Autodesk Fusion 360 part; units mm, degrees
note: some values were not read from the file. Chosen so that the rebuilt part matches the saved one: which face or edge a step refers to. Set by a fixed rule: which sketch regions a step uses; the direction of a hole.
(part 4 of 4)
sketch "Sketch157" plane through (150, 0, 0) normal (-1, 0, 0) x (0, -1, 0)
  line L0 (0, 69) -> (10, 69)
  line L1 (10, 69) -> (10, 66)
  line L2 (10, 66) -> (0, 66)
  line L3 (0, 66) -> (0, 0)
  line L4 (0, 0) -> (45, 0)
  line L5 (45, 0) -> (45, 66)
  line L6 (45, 66) -> (35, 66)
  line L7 (35, 66) -> (35, 69)
  line L8 (35, 69) -> (45, 69)
  line L9 (45, 69) -> (45, 75)
  line L10 (45, 75) -> (34, 75)
  line L11 (34, 75) -> (34, 80)
  line L12 (34, 80) -> (11, 80)
  line L13 (11, 80) -> (11, 75)
  line L14 (11, 75) -> (0, 75)
  line L15 (0, 75) -> (0, 69)
  line L16 (15, 33) -> (30, 33)
  line L17 (30, 33) -> (30, 27)
  line L18 (30, 27) -> (15, 27)
  line L19 (15, 27) -> (15, 33)
  circle A0 centre (17.9, 30) radius 1.5
  circle A1 centre (27.1, 30) radius 1.5
  dimension "d1193" = 27
  dimension "d1194" = 3
  dimension "d1195" = 3
  dimension "d1196" = 9.2
  dimension "d1197" = 3
  dimension "d1198" = 15
  dimension "d1199" = 2.9
  dimension "d1200" = 6
  constraint horizontal L16
  constraint vertical L17
  constraint horizontal L18
  constraint vertical L19
  measures "d1193" distance of L4 L18
  measures "d1194" diameter of A0
  measures "d1195" diameter of A1
  measures "d1196" distance of A0.centre A1.centre
  measures "d1197" distance of L18 A0.centre
  measures "d1198" distance of L16.start L16.end
  measures "d1199" distance of L19 A0.centre
  measures "d1200" distance of L16.start L18.end
extrude "Extrude200" add sketch "Sketch157" along normal blind 10 contours L16 L17 L18 L19 bodies 6
extrude "Extrude201" cut sketch "Sketch157" against normal blind 78.085 contours A0 | A1 bodies 6
sketch "Sketch158" plane through (170, 0, 0) normal (1, 0, 0) x (0, 1, 0)
  circle A0 centre (-17.9, 30) radius 1.5
  circle A1 centre (-27.1, 30) radius 1.5
  line L0 (0, 47) -> (-45, 47)
  line L1 (-45, 47) -> (-45, 10)
  line L2 (-45, 10) -> (0, 10)
  line L3 (0, 10) -> (0, 47)
  circle A2 centre (-27.1, 30) radius 3.5
  circle A3 centre (-17.9, 30) radius 3.5
  dimension "d1205" = 7
  dimension "d1206" = 7
  constraint concentric A1 A2
  constraint concentric A0 A3
  measures "d1205" diameter of A2
  measures "d1206" diameter of A3
extrude "Extrude202" cut sketch "Sketch158" against normal blind 3 contours A2 | A3 bodies 6
extrude "Extrude203" add 1 faces at (-154.4778, 172, 27.586) along direction (0, -1, 0) blind 2.2 on bodies 1 bodies 1
sketch "Sketch159" plane through (0, 0, 120) normal (0, 0, 1) x (-1, 0, 0)
  line L0 (175, -164.8202) -> (171.994, -164.8202)
  line L1 (171.994, -164.8202) -> (171.994, -165.8202)
  line L2 (171.994, -165.8202) -> (169.294, -165.8202)
  line L3 (169.294, -165.8202) -> (169.294, -164.8202)
  line L4 (169.294, -164.8202) -> (160, -164.8202)
  line L5 (160, -164.8202) -> (160, -174.8202)
  line L6 (160, -174.8202) -> (175, -174.8202)
  line L7 (175, -174.8202) -> (175, -164.8202)
  circle A0 centre (163.5, -171.3202) radius 1.5
  circle A1 centre (163.5, -108.3202) radius 1.5
  line L8 (175, -104.8202) -> (160, -104.8202)
  line L9 (160, -104.8202) -> (160, -114.8202)
  dimension "d1211" = 3
  dimension "d1212" = 3.5
  dimension "d1213" = 3.5
  dimension "d1214" = 3
  dimension "d1215" = 3.5
  dimension "d1216" = 3.5
  measures "d1211" diameter of A0
  measures "d1212" distance of L5 A0.centre
  measures "d1213" distance of L6 A0.centre
  measures "d1214" diameter of A1
  measures "d1215" distance of A1.centre L8
  measures "d1216" distance of A1.centre L9
extrude "Extrude204" cut sketch "Sketch159" against normal blind 35 contours A0 | A1 bodies 1
extrude "Extrude205" cut sketch "Sketch155" against normal blind 7 contours L10 L21 L22 L23 L24 | L7 L17 L18 L19 L20 bodies 1
sketch "Sketch160" plane through (0, 0, 15) normal (0, 0, 1) x (-1, 0, 0)
  line L0 (175, 4.7712) -> (25, 4.7712)
  line L1 (25, 4.7712) -> (25, 0)
  line L2 (25, 0) -> (-15, 0)
  line L3 (-15, 0) -> (-15, -30)
  line L4 (-15, -30) -> (190, -30)
  line L5 (190, -30) -> (190, -5)
  line L6 (190, -5) -> (176, -5)
  arc A0 (175, -4) -> (176, -5) centre (175, -5) ccw
  line L7 (175, -4) -> (175, 4.7712)
  circle A1 centre (120, -15) radius 2.5
  circle A2 centre (120, 75) radius 2.5
  circle A3 centre (55, 75) radius 2.5
  circle A4 centre (55, -15) radius 2.5
  circle A5 centre (120, 75) radius 5
  circle A6 centre (120, -15) radius 5
  circle A7 centre (55, -15) radius 5
  circle A8 centre (55, 75) radius 5
  line L8 (190, -30) -> (190, -10)
  line L9 (190, 65) -> (190, 90)
  line L10 (-15, 90) -> (-15, 60)
  line L11 (190, 90) -> (-15, 90)
  line L12 (-15, -30) -> (190, -30)
  dimension "d1227" = 5
  dimension "d1228" = 5
  dimension "d1229" = 5
  dimension "d1230" = 5
  dimension "d1235" = 70
  dimension "d1236" = 70
  dimension "d1237" = 70
  dimension "d1238" = 70
  dimension "d1239" = 15
  dimension "d1240" = 15
  dimension "d1241" = 15
  dimension "d1242" = 15
  constraint concentric A2 A5
  constraint concentric A1 A6
  constraint concentric A4 A7
  constraint concentric A3 A8
  measures "d1227" diameter of A1
  measures "d1228" diameter of A2
  measures "d1229" diameter of A3
  measures "d1230" diameter of A4
  measures "d1235" distance of A1.centre L8
  measures "d1236" distance of L3 A4.centre
  measures "d1237" distance of A2.centre L9
  measures "d1238" distance of A3.centre L10
  measures "d1239" distance of A3.centre L11
  measures "d1240" distance of A2.centre L11
  measures "d1241" distance of A1.centre L12
  measures "d1242" distance of A4.centre L12
extrude "Extrude206" cut sketch "Sketch160" against normal blind 22.636 contours A1 | A2 | A3 | A4 bodies 2
extrude "Extrude207" cut sketch "Sketch160" against normal blind 10 contours A5 | A6 | A7 | A8 bodies 2
sketch "Sketch161" plane through (0, 0, 0) normal (0, 0, 1) x (1, 0, 0)
  line L0 (-75, -100) -> (-160, -100)
  line L1 (-160, -100) -> (-160, -220)
  line L2 (-160, -220) -> (-75, -220)
  line L3 (-75, -220) -> (-75, -100)
  circle A0 centre (-150, -115) radius 2.5
  circle A1 centre (-85, -115) radius 2.5
  circle A2 centre (-150, -205) radius 2.5
  circle A3 centre (-85, -205) radius 2.5
  dimension "d1243" = 85
  dimension "d1244" = 120
  dimension "d1245" = 5
  dimension "d1246" = 5
  dimension "d1247" = 65
  dimension "d1248" = 5
  dimension "d1249" = 5
  dimension "d1250" = 65
  dimension "d1251" = 90
  dimension "d1252" = 15
  constraint horizontal L0
  constraint vertical L1
  constraint horizontal L2
  constraint vertical L3
  measures "d1243" distance of L0.start L0.end
  measures "d1244" distance of L0.start L2.end
  measures "d1245" diameter of A0
  measures "d1246" diameter of A1
  measures "d1247" distance of A0.centre A1.centre
  measures "d1248" diameter of A2
  measures "d1249" diameter of A3
  measures "d1250" distance of A2.centre A3.centre
  measures "d1251" distance of A1.centre A3.centre
  measures "d1252" distance of L2 A3.centre
extrude "Extrude208" add sketch "Sketch161" along normal blind 7 separate body makes body 12
sketch "Sketch163" plane through (0, 0, 7) normal (0, 0, 1) x (-1, 0, 0)
  circle A0 centre (150, 115) radius 2.5
  circle A1 centre (150, 205) radius 2.5
  circle A2 centre (85, 205) radius 2.5
  circle A3 centre (85, 115) radius 2.5
  line L0 (75, 220) -> (75, 100)
  line L1 (75, 100) -> (160, 100)
  line L2 (160, 100) -> (160, 220)
  line L3 (160, 220) -> (75, 220)
  line L4 (117.5, 160) -> (138.9, 160)
  line L5 (138.9, 160) -> (138.9, 138.8)
  line L6 (138.9, 138.8) -> (117.5, 138.8)
  line L7 (117.5, 138.8) -> (117.5, 160)
  line L8 (138.9, 138.8) -> (96.1, 138.8)
  line L9 (96.1, 138.8) -> (96.1, 181.2)
  line L10 (96.1, 181.2) -> (138.9, 181.2)
  line L11 (138.9, 181.2) -> (138.9, 138.8)
  dimension "d1263" = 21.4
  dimension "d1264" = 21.2
  dimension "d1265" = 42.8
  dimension "d1266" = 42.4
  constraint horizontal L4
  constraint vertical L5
  constraint horizontal L6
  constraint vertical L7
  constraint horizontal L8
  constraint vertical L9
  constraint horizontal L10
  constraint vertical L11
  measures "d1263" distance of L4.start L4.end
  measures "d1264" distance of L4.start L6.end
  measures "d1265" distance of L5.end L8.end
  measures "d1266" distance of L5.end L10.end
extrude "Extrude209" add sketch "Sketch163" along normal blind 9.5 contours L4 L7 L8 L9 L10 L11 | L4 L5 L6 L7 L8 L11 bodies 12
sketch "Sketch164" plane through (0, -181.2, 0) normal (0, -1, 0) x (1, 0, 0)
  line L0 (-138.9, 7) -> (-96.1, 7)
  line L1 (-96.1, 7) -> (-96.1, 16.5)
  line L2 (-96.1, 16.5) -> (-138.9, 16.5)
  line L3 (-138.9, 16.5) -> (-138.9, 7)
  line L4 (-138.9, 16.5) -> (-96.1, 16.5)
  line L5 (-96.1, 16.5) -> (-96.1, 13.5)
  line L6 (-96.1, 13.5) -> (-138.9, 13.5)
  line L7 (-138.9, 13.5) -> (-138.9, 16.5)
  dimension "d1269" = 3
  constraint horizontal L4
  constraint vertical L5
  constraint horizontal L6
  constraint vertical L7
  constraint coincident L1 L5.end
  constraint coincident L2.end L3.start
  measures "d1269" distance of L2.end L6.end
extrude "Extrude210" cut sketch "Sketch164" against normal blind 0.01 contours L0 L1 L3 L6 bodies 12
sketch "Sketch165" plane through (-96.1, 0, 0) normal (1, 0, 0) x (0, 1, 0)
  line L0 (-181.2, 13.5) -> (-181.19, 13.5)
  line L1 (-181.19, 13.5) -> (-181.19, 7)
  line L2 (-181.19, 7) -> (-138.8, 7)
  line L3 (-138.8, 7) -> (-138.8, 16.5)
  line L4 (-138.8, 16.5) -> (-181.2, 16.5)
  line L5 (-181.2, 16.5) -> (-181.2, 13.5)
  line L6 (-181.19, 13.5) -> (-138.8, 13.5)
  line L7 (-138.8, 13.5) -> (-138.8, 16.5)
  line L8 (-138.8, 16.5) -> (-181.19, 16.5)
  line L9 (-181.19, 16.5) -> (-181.19, 13.5)
  constraint horizontal L6
  constraint vertical L7
  constraint horizontal L8
  constraint vertical L9
  constraint coincident L3.end L4.start
  constraint coincident L0.end L1.start
sketch "Sketch166" plane through (0, -138.8, 0) normal (0, 1, 0) x (-1, 0, 0)
  line L0 (96.1, 7) -> (138.9, 7)
  line L1 (138.9, 7) -> (138.9, 16.5)
  line L2 (138.9, 16.5) -> (96.1, 16.5)
  line L3 (96.1, 16.5) -> (96.1, 7)
  line L4 (96.1, 16.5) -> (138.9, 16.5)
  line L5 (138.9, 16.5) -> (138.9, 13.5)
  line L6 (138.9, 13.5) -> (96.1, 13.5)
  line L7 (96.1, 13.5) -> (96.1, 16.5)
  dimension "d1272" = 3
  constraint horizontal L4
  constraint vertical L5
  constraint horizontal L6
  constraint vertical L7
  constraint coincident L2.end L3.start
  measures "d1272" distance of L2.end L6.end
sketch "Sketch167" plane through (-138.9, 0, 0) normal (-1, 0, 0) x (0, -1, 0)
  line L0 (181.19, 7) -> (181.19, 13.5)
  line L1 (181.19, 13.5) -> (181.2, 13.5)
  line L2 (181.2, 13.5) -> (181.2, 16.5)
  line L3 (181.2, 16.5) -> (138.8, 16.5)
  line L4 (138.8, 16.5) -> (138.8, 7)
  line L5 (138.8, 7) -> (181.19, 7)
  line L6 (138.8, 13.5156) -> (181.2, 13.5156)
  line L7 (181.2, 13.5156) -> (181.2, 16.5156)
  line L8 (181.2, 16.5156) -> (138.8, 16.5156)
  line L9 (138.8, 16.5156) -> (138.8, 13.5156)
  dimension "d1273" = 3
  constraint horizontal L6
  constraint vertical L7
  constraint horizontal L8
  constraint vertical L9
  constraint coincident L2 L7.end
  constraint coincident L4 L6.start
  measures "d1273" distance of L6.start L8.end
extrude "Extrude211" cut sketch "Sketch167" against normal blind 0.01 contours L0 L1 L2 L4 L5 L6 bodies 12
extrude "Extrude212" cut sketch "Sketch166" against normal blind 0.01 contours L0 L1 L3 L6 bodies 12
extrude "Extrude213" cut sketch "Sketch165" against normal blind 0.01 contours L1 L2 L3 L6 bodies 12
draft "Draft1" angle -18 neutral plane through (0, 0, 16.5) pull (0, 0, 1) 4 faces at (-110.37, -138.81, 11.3333) (-138.89, -152.9367, 9.1667) (-124.63, -181.19, 11.3333) (-96.11, -167.0633, 9.1667) on bodies 12
sketch "Sketch168" plane through (0, 0, 0) normal (0, 0, 1) x (1, 0, 0)
  line L0 (-225, 100) -> (-210, 100)
  line L1 (-210, 100) -> (-210, 30)
  line L2 (-210, 30) -> (-225, 30)
  line L3 (-225, 30) -> (-225, 100)
  circle A0 centre (-213.5, 33.5) radius 1.5
  circle A1 centre (-213.5, 96.5) radius 1.5
  dimension "d1282" = 3
  dimension "d1283" = 3
  dimension "d1284" = 3.5
  dimension "d1285" = 3.5
  dimension "d1286" = 3.5
  dimension "d1287" = 3.5
  constraint horizontal L0
  constraint vertical L1
  constraint horizontal L2
  constraint vertical L3
  measures "d1282" diameter of A0
  measures "d1283" diameter of A1
  measures "d1284" distance of L1 A1.centre
  measures "d1285" distance of L0 A1.centre
  measures "d1286" distance of L1 A0.centre
  measures "d1287" distance of L2 A0.centre
extrude "Extrude214" add sketch "Sketch168" along normal blind 30 separate body makes body 13
sketch "Sketch169" plane through (-225, 0, 0) normal (-1, 0, 0) x (0, -1, 0)
  line L0 (-100, 0) -> (-30, 0)
  line L1 (-30, 0) -> (-30, 30)
  line L2 (-30, 30) -> (-100, 30)
  line L3 (-100, 30) -> (-100, 0)
  circle A0 centre (-65, 30) radius 25
  circle A1 centre (-65, 0) radius 2.85
  circle A2 centre (-65, 0) radius 5
  line L4 (-75, 0) -> (-55, 0)
  dimension "d1290" = 50
  dimension "d1298" = 5.7
  dimension "d1318" = 20
  constraint midpoint L2 A0.centre
  constraint midpoint L0 A1.centre
  constraint concentric A1 A2
  constraint horizontal L4
  constraint coincident L0 L4.start
  measures "d1290" diameter of A0
  measures "d1298" diameter of A1
  measures "d1318" distance of L4.start L4.end
extrude "Extrude215" cut sketch "Sketch169" against normal blind 25.387 contours L2 A0 picked at (-70.4572, 23.7021) bodies 13
sketch "Sketch170" plane through (-221.994, 0, 0) normal (-1, 0, 0) x (0, -1, 0)
  line L0 (-90, 30) -> (-100, 30)
  line L1 (-100, 30) -> (-100, 0)
  line L2 (-100, 0) -> (-30, 0)
  line L3 (-30, 0) -> (-30, 30)
  line L4 (-30, 30) -> (-40, 30)
  arc A0 (-90, 30) -> (-40, 30) centre (-65, 30) ccw
  circle A1 centre (-65, 30) radius 26
  dimension "d1295" = 52
  constraint concentric A0 A1
  measures "d1295" diameter of A1
extrude "Extrude217" cut sketch "Sketch170" against normal blind 2.7 contours L0 L4 A0 A1 picked at (-90.5699, 28.7083) bodies 13
sketch "Sketch173" plane through (-210, 0, 0) normal (1, 0, 0) x (0, 1, 0)
  line L0 (30, 0) -> (100, 0)
  line L1 (100, 0) -> (100, 30)
  line L2 (100, 30) -> (90, 30)
  arc A0 (40, 30) -> (90, 30) centre (65, 30) ccw
  line L3 (40, 30) -> (30, 30)
  line L4 (30, 30) -> (30, 0)
  circle A1 centre (65, 0) radius 3.5
  line L5 (100, 30) -> (110, 30)
  line L6 (110, 20) -> (100, 20)
  line L7 (100, 20) -> (100, 30)
  circle A2 centre (110, 25) radius 5
  line L8 (108, 25) -> (105, 27.5)
  line L9 (105, 27.5) -> (100, 27.5)
  line L10 (108, 25) -> (105, 22.5)
  line L11 (105, 22.5) -> (100, 22.5)
  line L12 (30, 30) -> (20, 30)
  line L13 (20, 30) -> (20, 20)
  line L14 (20, 20) -> (30, 20)
  line L15 (30, 20) -> (30, 30)
  circle A3 centre (20, 25) radius 5
  line L16 (30, 25) -> (25, 25)
  line L17 (30, 25) -> (30, 27)
  line L18 (24.5826, 27) -> (30, 27)
  line L19 (30, 25) -> (30, 23)
  line L20 (24.5826, 23) -> (30, 23)
  circle A4 centre (20, 25) radius 3
  line L21 (107.5, 15) -> (112.6605, 15)
  line L22 (107.5, 15) -> (100, 15)
  line L23 (110, 23) -> (107.5, 20)
  line L24 (110, 23) -> (112.5, 20)
  line L25 (112.5, 20) -> (112.5, 15)
  line L26 (105, 27.5) -> (105, 30)
  line L27 (105, 22.5) -> (105, 20)
  dimension "d1343" = 10
  dimension "d1344" = 10
  constraint horizontal L5
  constraint horizontal L6
  constraint vertical L7
  constraint coincident L1.end L2.start
  constraint coincident L6.start A2
  constraint coincident L7 L9.end
  constraint coincident L7 L11.end
  constraint horizontal L12
  constraint vertical L13
  constraint horizontal L14
  constraint vertical L15
  constraint coincident L3.end L4.start
  constraint midpoint L13 A3.centre
  constraint coincident L12.end A3
  constraint midpoint L15 L16.start
  constraint coincident A3 L16.end
  constraint perpendicular L15 L16
  constraint coincident L15 L17.end
  constraint coincident A3 L18.start
  constraint perpendicular L15 L18
  constraint coincident L15 L19.end
  constraint coincident A3 L20.start
  constraint perpendicular L15 L20
  constraint concentric A3 A4
  constraint midpoint L1 L22.end
  constraint coincident L6 L23.end
  constraint coincident L21 L25.end
  constraint perpendicular L21 L25
  constraint midpoint L5 L26.end
  constraint midpoint L6 L27.end
  measures "d1343" distance of L3.end L12.end
  measures "d1344" distance of L3.end L14.end
move_body "Align1" bodies 1 to x (1, 0, 0) y (0, 1, 0) z (0, 0, 1) at (-14.5, -169.8202, 7)
extrude "Extrude221" add sketch "Sketch173" against normal blind 15 contours L1 L6 A2 L21 L22 L24 L25 | L1 L7 A2 L8 L9 L10 L11 | L4 L15 A3 L16 L19 L20 | L13 A3 A4 | L13 A3 A4 | L6 A2 L23 | L4 L15 A3 L16 L17 L18 | A2 L8 L10 | A2 L23 L24 bodies 13
move_body "Align11" bodies 3 to x (-1, 0, 0) y (0, -1, 0) z (0, 0, 1) at (-155, 110.0018, 15)
move_body "Align12" bodies 5 to x (1, 0, 0) y (0, 1, 0) z (0, 0, 1) at (-180, -7.4982, 40)
move_body "Align13" bodies 4 to x (1, 0, 0) y (0, 1, 0) z (0, 0, 1) at (-45, -334.9982, 40)
move_body "Move4" bodies 5 to x (1, 0, 0) y (0, 1, 0) z (0, 0, 1) at (0, 43.8306, 0)
move_body "Align14" bodies 13 to x (1, 0, 0) y (0, -1, 0) z (0, 0, -1) at (35.5, 35, 157)
sketch "Sketch179" plane through (0, 0, 63) normal (0, 0, 1) x (-1, 0, 0)
  line L0 (84.4696, 109.9982) -> (84.5133, 105.0379)
  arc A0 (75.9016, 103.17) -> (84.5133, 105.0379) centre (80.0135, 104.9982) ccw
  line L1 (75.9016, 103.17) -> (75.0135, 103.17)
  line L2 (75.0135, 103.17) -> (75.0135, 102.4982)
  arc A1 (75.0135, 102.4982) -> (77.5135, 99.9982) centre (77.5135, 102.4982) ccw
  line L3 (77.5135, 99.9982) -> (78.0135, 99.9982)
  line L4 (78.0135, 99.9982) -> (78.0135, 23.9982)
  line L5 (78.0135, 23.9982) -> (83.0135, 23.9982)
  line L6 (83.0135, 23.9982) -> (83.0135, 99.9982)
  line L7 (83.0135, 99.9982) -> (122.5135, 99.9982)
  arc A2 (122.5135, 99.9982) -> (125.0135, 102.4982) centre (122.5135, 102.4982) ccw
  line L8 (125.0135, 102.4982) -> (125.0135, 103.17)
  line L9 (125.0135, 103.17) -> (124.1119, 103.17)
  arc A3 (115.5, 104.9982) -> (124.1119, 103.17) centre (120, 104.9982) ccw
  line L10 (115.5, 104.9982) -> (115.5, 109.9982)
  line L11 (115.5, 109.9982) -> (84.4696, 109.9982)
  line L12 (95, 109.9982) -> (100.1112, 109.9982)
  line L13 (100.1112, 109.9982) -> (100.1112, 104.9964)
  line L14 (100.1112, 104.9964) -> (95, 104.9964)
  line L15 (95, 104.9964) -> (95, 109.9982)
  constraint horizontal L12
  constraint vertical L13
  constraint horizontal L14
  constraint vertical L15
  constraint coincident L11 L12.end
extrude "Extrude226" add sketch "Sketch179" along normal blind 71.5 contours L11 L12 L13 L14 L15 bodies 4
sketch "Sketch180" plane through (-95, 0, 0) normal (1, 0, 0) x (0, 1, 0)
  line L0 (-109.9982, 63) -> (-104.9964, 63)
  line L1 (-104.9964, 63) -> (-104.9964, 134.5)
  line L2 (-104.9964, 134.5) -> (-109.9982, 134.5)
  line L3 (-109.9982, 134.5) -> (-109.9982, 63)
  line L4 (-77, 132) -> (-80, 134.5)
  line L5 (-80, 134.5) -> (-104.9964, 134.5)
  line L6 (-77, 132) -> (-80, 129.5)
  line L7 (-80, 129.5) -> (-104.9964, 129.5)
  circle A0 centre (-86.3524, 110.856) radius 18.644
  circle A1 centre (-75, 132) radius 6
  circle A2 centre (-75, 132) radius 8
  line L8 (-75, 127) -> (-77.5, 127)
  line L9 (-75, 127) -> (-72.5, 127)
  line L10 (-72.5, 127) -> (-72.5, 126.5456)
  line L11 (-77.5, 127) -> (-77.5, 126.5456)
  line L12 (-75, 130) -> (-77.5, 127)
  line L13 (-75, 130) -> (-72.5, 127)
  dimension "d1342" = 5
  dimension "d1345" = 2.5
  dimension "d1346" = 2.5
  constraint coincident L1 L2.start
  constraint perpendicular L1 L5
  constraint coincident L1 L7.end
  constraint perpendicular L1 L7
  constraint tangent L7 A0
  constraint tangent L1 A0
  constraint concentric A1 A2
  constraint horizontal L8
  constraint parallel L8 L9
  constraint coincident A1 L10.end
  constraint perpendicular L9 L10
  constraint coincident A1 L11.end
  constraint perpendicular L8 L11
  measures "d1342" distance of L5 L7
  measures "d1345" distance of L8.start L8.end
  measures "d1346" distance of L8.start L9.end
extrude "Extrude227" add sketch "Sketch180" against normal blind 5 contours L0 L1 L2 L3 | L1 L7 A0 | L1 L5 L7 A2 | L5 A0 A1 A2 | L5 L7 A1 A2 | L7 A0 A1 A2 | A0 A1 A2 | L4 L5 L6 L7 A1 | A0 A1 L8 L11 | A0 A1 L8 L9 L10 | A0 L8 L9 L12 L13 | A0 L8 L12 bodies 4
equation "d913 = 42.3 mm + 20 mm + 20 mm"
equation "d937 = 42.3 mm + 20 mm + 20 mm"
equation "d973 = 15 mm + 55 mm - 3 mm"
equation "d990 = 11 mm + 30 mm"
equation "d1070 = 10 mm + 5 mm"
equation "d1139 = 3 mm + ( 2 * 0.85 ) * 1 mm"
equation "d1141 = 0.85 mm + 1.5 mm"
equation "d1190 = ( 4 * 2 ) * 1 mm + 9.5 mm"
equation "d1199 = ( ( 15 - 9.2 ) / 2 ) * 1 mm"
